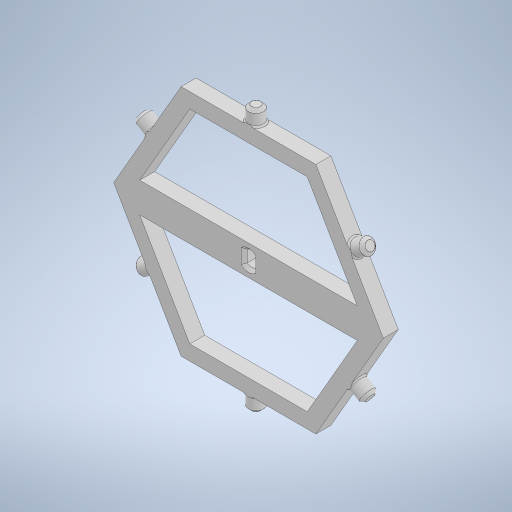
# Autodesk Inventor part: inner_bottom
Saved by Autodesk Inventor 2024 (Build 280153000, 153)
## iProperties
Created: 2024-03-21
Part Number: inner_bottom
Material: 일반
Document SubType Name: Modeling
Designer: SSAFY
Density: 1 g/cm^3
Appearance: 기본값
Author: SSAFY
Autodesk Inventor part; units mm, degrees
ref_plane "YZ Plane" through (0, 0, 0) normal (1, 0, 0) x (0, 1, 0)
ref_plane "XZ Plane" through (0, 0, 0) normal (0, 1, 0) x (-1, 0, 0)
ref_plane "XY Plane" through (0, 0, 0) normal (0, 0, 1) x (1, 0, 0)
sketch "스케치1" plane through (0, 0, 0) normal (0, 0, 1) x (1, 0, 0)
  line L0 (-45, 0) -> (-22.5, 38.971143)
  line L1 (-22.5, 38.971143) -> (22.5, 38.971143)
  line L2 (22.5, 38.971143) -> (45, 0)
  line L3 (45, 0) -> (22.5, -38.971143)
  line L4 (22.5, -38.971143) -> (-22.5, -38.971143)
  line L5 (-22.5, -38.971143) -> (-45, 0)
  line L6 (-19.613249, 33.971143) -> (-39.226497, 0)
  line L7 (-39.226497, 0) -> (-19.613249, -33.971143)
  line L8 (-19.613249, -33.971143) -> (19.613249, -33.971143)
  line L9 (19.613249, -33.971143) -> (39.226497, 0)
  line L10 (39.226497, 0) -> (19.613249, 33.971143)
  line L11 (19.613249, 33.971143) -> (-19.613249, 33.971143)
  line L12 (-42.113249, 5) -> (42.113249, 5)
  line L13 (-42.113249, -5) -> (42.113249, -5)
  circle A0 centre (0, 0) radius 2.5
  line L14 (-1.5, 2) -> (-1.5, -2)
  line L15 (1.5, 2) -> (1.5, -2)
  point P0 (36.339746, -5)
  point P1 (-36.339746, -5)
  point P2 (36.339746, 5)
  point P3 (-36.339746, 5)
  dimension "d0" = 45
  dimension "d1" = 5
  dimension "d2" = 5
  dimension "d3" = 5
  dimension "d4" = 5
  dimension "d5" = 3
  dimension "d6" = 1.5
  constraints: 32 end point, 4 point on circle, 4 point on line, 2 coincident, 2 parallel, 1 centre point, 1 horizontal, 1 vertical, 18 other
  measures "d0" distance of L0.end L1.end
  measures "d1" distance between parallel lines of L6 L0
  measures "d2" distance from line of L13 point (0, 0)
  measures "d3" distance from line of point (0, 0) L12
  measures "d4" diameter of A0
  measures "d5" distance between parallel lines of L15 L14
  measures "d6" distance from line of L15 point (0, 0)
extrude "돌출1" add sketch "스케치1" along normal blind 5 contours L0 L12 L6 L7 L13 L5 | L0 L1 L2 L12 L10 L11 L6 | L13 L7 L8 L9 L3 L4 L5 | L12 L10 L9 L13 L7 L6 | L12 L2 L3 L13 L9 L10 | A0 L15 | L14 A0
sketch "스케치2" plane through (-22.5, 38.971143, 0) normal (0, 1, 0) x (1, 0, 0)
  line L0 (45, 0) -> (0, 0) construction
  circle A0 centre (22.5, -2.5) radius 2.5
  point P0 (22.5, 0)
  dimension "d9" = 5
  constraints: 1 centre point, 1 tangent
  measures "d9" diameter of A0
extrude "돌출2" add sketch "스케치2" along normal blind 5
chamfer "모따기1" distance 1 angle 45 1 edges at (-2.5, 43.9711, 2.5)
pattern_circular "원형 패턴1" count 6 over 360 about axis through (0, 0, -10) along (0, 0, 1) of "돌출2", "모따기1"
chamfer "모따기2" distance 0.5 angle 45 18 edges at (1.7678, 38.9711, 0.7322) (1.7678, 38.9711, 4.2678) (-2.5, 38.9711, 2.5) (34.6339, 17.9546, 4.2678) (34.6339, 17.9546, 0.7322) (32.5, 21.6506, 2.5) (35, -17.3205, 2.5) (32.8661, -21.0165, 0.7322) (32.8661, -21.0165, 4.2678) (2.5, -38.9711, 2.5) (-1.7678, -38.9711, 0.7322) (-1.7678, -38.9711, 4.2678) (-32.5, -21.6506, 2.5) (-34.6339, -17.9546, 0.7322) (-34.6339, -17.9546, 4.2678) (-35, 17.3205, 2.5) (-32.8661, 21.0165, 0.7322) (-32.8661, 21.0165, 4.2678)
chamfer "모따기3" distance 1 angle 45 4 edges at (-1.5, 0, 5) (0, 2.5, 5) (1.5, 0, 5) (0, -2.5, 5)
